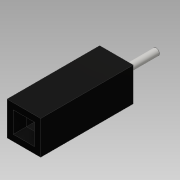
# Autodesk Inventor part: Pin-round-2.54-female
Saved by Autodesk Inventor 2016 (Build 200138000, 138)
## iProperties
Created: 2016-05-26
Part Number: Pin-round-2.54-female
Material: Generic
Document SubType Name: Modeling
Designer: admin
Density: 1 g/cm^3
Appearance: Default
Author: admin
Autodesk Inventor part; units mm, degrees
ref_plane "YZ Plane" through (0, 0, 0) normal (1, 0, 0) x (0, 1, 0)
ref_plane "XZ Plane" through (0, 0, 0) normal (0, 1, 0) x (-1, 0, 0)
ref_plane "XY Plane" through (0, 0, 0) normal (0, 0, 1) x (1, 0, 0)
sketch "Sketch1" plane through (0, 0, 0) normal (0, 1, 0) x (-1, 0, 0)
  line L0 (1.27, -1.27) -> (-1.27, -1.27)
  line L1 (-1.27, -1.27) -> (-1.27, 1.27)
  line L2 (-1.27, 1.27) -> (1.27, 1.27)
  line L3 (1.27, 1.27) -> (1.27, -1.27)
  point P0 (0, 0)
  point P1 (0, -1.27)
  point P2 (1.27, 0)
  dimension "d2" = 2.54
  constraints: 8 end point, 2 midpoint, 2 parallel, 2 perpendicular, 1 horizontal, 1 horizontal alignment, 1 vertical alignment
  measures "d2" distance between parallel lines of L2 L0
extrude "Extrusion1" add sketch "Sketch1" along normal blind 7
sketch "Sketch6" plane through (0, 7, 0) normal (0, 1, 0) x (1, 0, 0)
  circle A0 centre (0, 0) radius 0.25
  dimension "d19" = 0.5
  constraints: 1 centre point, 1 coincident
  measures "d19" diameter of A0
sketch "Sketch7" plane through (0, 0, 0) normal (0, -1, 0) x (1, 0, 0)
  line L0 (-0.3, 0.3) -> (0.3, 0.3)
  line L1 (0.3, 0.3) -> (0.3, -0.3)
  line L2 (0.3, -0.3) -> (-0.3, -0.3)
  line L3 (-0.3, -0.3) -> (-0.3, 0.3)
  point P0 (0, 0)
  point P1 (0, 0.3)
  point P2 (-0.3, 0)
  dimension "d20" = 0.6
  constraints: 8 end point, 2 midpoint, 2 parallel, 2 perpendicular, 1 horizontal, 1 horizontal alignment, 1 vertical alignment
  measures "d20" distance of L1.end L2.end
extrude "Extrusion4" cut sketch "Sketch7" against normal blind 5
chamfer "Chamfer1" distance 0.5 angle 45 4 edges at (0, 0, 0.3) (0.3, 0, 0) (0, 0, -0.3) (-0.3, 0, 0)
extrude "Extrusion5" add sketch "Sketch6" along normal blind 3
body "Solid1"
